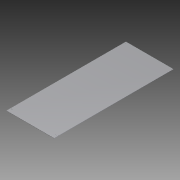
# Autodesk Inventor part: Base Top
Saved by Autodesk Inventor 2012 (Build 160160000, 160)
## iProperties
Created: 2011-10-13
Part Number: Base Top
Material: Default
Document SubType Name: Sheet Metal
Designer: Tushar
Density: 1 g/cm^3
Sheet Metal Rule: Default
Author: Tushar
Autodesk Inventor part; units mm, degrees
ref_plane "YZ Plane" through (0, 0, 0) normal (1, 0, 0) x (0, 1, 0)
ref_plane "XZ Plane" through (0, 0, 0) normal (0, 1, 0) x (-1, 0, 0)
ref_plane "XY Plane" through (0, 0, 0) normal (0, 0, 1) x (1, 0, 0)
sketch "Sketch2" plane through (0, 0, 0) normal (0, 1, 0) x (-1, 0, 0)
  line L0 (-301.752, -756.8438) -> (301.752, -756.8438)
  line L1 (301.752, -756.8438) -> (301.752, 756.8438)
  line L2 (301.752, 756.8438) -> (-301.752, 756.8438)
  line L3 (-301.752, 756.8438) -> (-301.752, -756.8438)
  point P0 (0, 0)
  dimension "d0" = 301.752
  dimension "d1" = 301.752
  dimension "d2" = 756.8438
  dimension "d3" = 756.8438
  measures "d0" distance from line of L1 point (0, 0)
  measures "d1" distance from line of L3 point (0, 0)
  measures "d2" distance from line of L0 point (0, 0)
  measures "d3" distance from line of L2 point (0, 0)
extrude "Plate1" add sketch "Sketch2" along normal blind 3.048
sketch "Sketch3" plane through (0, 3.048, 0) normal (0, 1, 0) x (1, 0, 0)
  line L0 (301.752, 756.8438) -> (301.752, -756.8438) projected
  line L1 (-301.752, -756.8438) -> (-301.752, 756.8438) projected
  line L2 (301.752, -756.8438) -> (-301.752, -756.8438) projected
  point P0 (0, 0)
  point P1 (-295.529, -698.9572)
  point P2 (276.479, -698.9572)
  dimension "d5" = 6.223
  dimension "d6" = 25.273
  dimension "d22" = 57.8866
  dimension "d23" = 57.8866
  measures "d5" distance from line of L1 point (-295.529, -698.957)
  measures "d6" distance from line of L0 point (276.479, -698.957)
  measures "d22" distance from line of L2 point (-295.529, -698.957)
  measures "d23" distance from line of L2 point (276.479, -698.957)
hole "Hole1" at (-295.529, 3.048, 698.9572) at (276.479, 3.048, 698.9572) direction (0, -1, 0) diameter 3.175 end through all
sketch "Sketch4" plane through (0, 3.048, 0) normal (0, 1, 0) x (1, 0, 0)
  circle A0 centre (-295.529, -698.9572) radius 1.5875 projected
  line L0 (301.752, -756.8438) -> (-301.752, -756.8438) projected
  line L1 (-295.529, -698.9572) -> (-270.8654, -698.9572)
  point P0 (0, 0)
  constraints: 2 end point, 1 parallel
sketch "Sketch5" plane through (0, 3.048, 0) normal (0, 1, 0) x (1, 0, 0)
  circle A0 centre (-295.529, -698.9572) radius 1.5875 projected
  line L0 (301.752, -756.8438) -> (-301.752, -756.8438) projected
  line L1 (-295.529, -698.9572) -> (-295.529, -717.14)
  line L2 (301.752, 756.8438) -> (301.752, -756.8438) projected
  point P0 (0, 0)
  constraints: 2 end point, 1 parallel, 1 perpendicular
pattern_linear "Rectangular Pattern1" count 3 spacing 9.525 along (1, 0, 0) count 2 spacing 9.525 along (0, 0, 1) of "Hole1"
sketch "Sketch6" plane through (0, 3.048, 0) normal (0, 1, 0) x (1, 0, 0)
  line L0 (301.752, 756.8438) -> (301.752, -756.8438) projected
  line L1 (-301.752, 756.8438) -> (301.752, 756.8438) projected
  line L2 (-301.752, -756.8438) -> (-301.752, 756.8438) projected
  point P0 (0, 0)
  point P1 (291.084, 750.4938)
  point P2 (286.639, 744.1438)
  point P3 (291.084, 737.7938)
  point P4 (286.639, 731.4438)
  point P5 (-291.084, 750.4938)
  point P6 (-286.639, 744.1438)
  point P7 (-291.084, 737.7938)
  point P8 (-286.639, 731.4438)
  dimension "d24" = 10.668
  dimension "d25" = 4.445
  dimension "d26" = 6.35
  dimension "d27" = 6.35
  dimension "d28" = 6.35
  dimension "d29" = 6.35
  dimension "d30" = 10.668
  dimension "d31" = 4.445
  constraints: 4 horizontal alignment, 4 vertical alignment
  measures "d24" distance from line of L0 point (291.084, 750.494)
  measures "d25" horizontal distance of point (291.084, 750.494) point (286.639, 744.144)
  measures "d26" vertical distance of point (286.639, 744.144) point (291.084, 750.494)
  measures "d27" distance from line of point (291.084, 750.494) L1
  measures "d28" vertical distance of point (291.084, 737.794) point (286.639, 744.144)
  measures "d29" vertical distance of point (286.639, 731.444) point (291.084, 737.794)
  measures "d30" distance from line of L2 point (-291.084, 750.494)
  measures "d31" horizontal distance of point (-286.639, 744.144) point (-291.084, 750.494)
hole "Hole2" at (291.084, 3.048, -750.4938) at (286.639, 3.048, -744.1438) at (291.084, 3.048, -737.7938) at (286.639, 3.048, -731.4438) at (-291.084, 3.048, -750.4938) at (-286.639, 3.048, -744.1438) at (-291.084, 3.048, -737.7938) at (-286.639, 3.048, -731.4438) direction (0, -1, 0) diameter 3.175 end through all
equation "\"d23\" = d22"
equation "\"d14\" = Thickness"
equation "\"d37\" = Thickness"
equation "\"d1\" = d0"
equation "\"d3\" = d2"
equation "\"BendRadius\" = Thickness"
equation "\"BendReliefWidth\" = Thickness"
equation "\"BendReliefDepth\" = 0.5 * Thickness"
equation "\"CornerReliefSize\" = 4 * Thickness"
equation "\"MinimumRemnant\" = 2 * Thickness"
equation "\"TransitionRadius\" = BendRadius"
equation "\"JacobiRadiusSize\" = BendRadius"
equation "\"GapSize\" = Thickness"
equation "\"d4\" = BendRadius"
equation "\"Thickness\" = 3.048"
body "Solid1"
